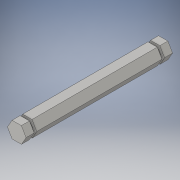
# Autodesk Inventor part: Shafts
Saved by Autodesk Inventor 2016 (Build 200138000, 138)
## iProperties
Created: 2016-02-01
Part Number: Shafts
Material: Generic
Document SubType Name: Modeling
Designer: Mentor1102
Density: 1 g/cm^3
Appearance: Default
Author: Mentor1102
Autodesk Inventor part; units mm, degrees
ref_plane "YZ Plane" through (0, 0, 0) normal (1, 0, 0) x (0, 1, 0)
ref_plane "XZ Plane" through (0, 0, 0) normal (0, 1, 0) x (-1, 0, 0)
ref_plane "XY Plane" through (0, 0, 0) normal (0, 0, 1) x (1, 0, 0)
sketch "Sketch1" plane through (0, 0, 0) normal (0, 0, 1) x (1, 0, 0)
  line L0 (3.634, 6.3685) -> (7.3323, 0.0371)
  line L1 (7.3323, 0.0371) -> (3.6983, -6.3314)
  line L2 (3.6983, -6.3314) -> (-3.634, -6.3685)
  line L3 (-3.634, -6.3685) -> (-7.3323, -0.0371)
  line L4 (-7.3323, -0.0371) -> (-3.6983, 6.3314)
  line L5 (-3.6983, 6.3314) -> (3.634, 6.3685)
  point P0 (0, 0)
  point P1 (0, 0)
  dimension "d0" = 12.7
  constraints: 12 end point, 1 coincident, 13 other
  measures "d0" distance between parallel lines of L2 L5
extrude "Extrusion1" add sketch "Sketch1" along normal blind 98.5266
sketch "Sketch2" plane through (0, 0, 98.5266) normal (0, 0, 1) x (1, 0, 0)
  circle A0 centre (0, 0) radius 4.191
  dimension "d3" = 8.382
  constraints: 1 centre point, 1 coincident
  measures "d3" diameter of A0
extrude "Extrusion2" add sketch "Sketch2" along normal blind 2
sketch "Sketch3" plane through (0, 0, 0) normal (0, 0, -1) x (-1, 0, 0)
  circle A0 centre (0, 0) radius 4.191
  dimension "d6" = 8.382
  constraints: 1 centre point, 1 coincident
  measures "d6" diameter of A0
extrude "Extrusion3" add sketch "Sketch3" along normal blind 2
sketch "Sketch4" plane through (0, 0, 100.5266) normal (0, 0, 1) x (1, 0, 0)
  circle A0 centre (0, 0) radius 4.191 construction
  line L0 (7.3323, 0.0371) -> (3.634, 6.3685) projected
  line L1 (3.634, 6.3685) -> (-3.6983, 6.3314) projected
  line L2 (-3.6983, 6.3314) -> (-7.3323, -0.0371) projected
  line L3 (-7.3323, -0.0371) -> (-3.634, -6.3685) projected
  line L4 (-3.634, -6.3685) -> (3.6983, -6.3314) projected
  line L5 (3.6983, -6.3314) -> (7.3323, 0.0371) projected
extrude "Extrusion4" add sketch "Sketch4" along normal blind 6.35
sketch "Sketch5" plane through (0, 0, -2) normal (0, 0, -1) x (-1, 0, 0)
  circle A0 centre (0, 0) radius 4.191 construction
  line L0 (-3.634, 6.3685) -> (-7.3323, 0.0371) projected
  line L1 (-7.3323, 0.0371) -> (-3.6983, -6.3314) projected
  line L2 (-3.6983, -6.3314) -> (3.634, -6.3685) projected
  line L3 (3.634, -6.3685) -> (7.3323, -0.0371) projected
  line L4 (7.3323, -0.0371) -> (3.6983, 6.3314) projected
  line L5 (3.6983, 6.3314) -> (-3.634, 6.3685) projected
extrude "Extrusion5" add sketch "Sketch5" along normal blind 6.35
body "Solid1"
